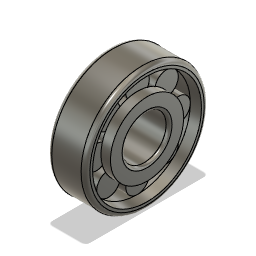
Bearing_GOST_8328-75_12000 (Autodesk Fusion 360 design; units mm, degrees)
Autodesk Fusion 360 part; units mm, degrees
sketch "Sketch1" plane through (0, 0, 0) normal (0, 0, 1) x (1, 0, 0)
  line L0 (-41.4222, 0) -> (41.4222, 0)
  line L1 (-6.5, 7.5) -> (6.5, 7.5)
  line L2 (6.5, 7.5) -> (6.5, 12.4792)
  line L3 (6.5, 12.4792) -> (3.25, 12.4792)
  line L4 (3.25, 12.4792) -> (3.25, 10)
  line L5 (3.25, 10) -> (-3.25, 10)
  line L6 (-3.25, 10) -> (-3.25, 12.4792)
  line L7 (-3.25, 12.4792) -> (-6.5, 12.4792)
  line L8 (-6.5, 12.4792) -> (-6.5, 7.5)
  line L9 (-6.5, 16.5) -> (-6.5, 21)
  line L10 (-6.5, 21) -> (6.5, 21)
  line L11 (6.5, 21) -> (6.5, 18.5731)
  line L12 (6.5, 18.5731) -> (3.25, 18)
  line L13 (3.25, 18) -> (-3.25, 18)
  line L14 (-3.25, 18) -> (-3.25, 16.5)
  line L15 (-3.25, 16.5) -> (-6.5, 16.5)
  line L16 (-3.25, 16.5) -> (-3.25, 12.4792)
  line L17 (3.25, 18) -> (3.25, 12.4792)
  line L18 (0, 18) -> (0, 10) construction
  line L19 (-3.25, 14) -> (3.25, 14)
  point P0 (0, 7.5)
  point P1 (0, 14)
  dimension "d1" = 15
  dimension "d2" = 13
  dimension "d3" = 10
  dimension "d4" = 42
  dimension "d5" = 3.25
  dimension "d6" = 24.9585
  dimension "d7" = 20
  dimension "d8" = 33
  dimension "d9" = 36
  constraint horizontal L0
  constraint midpoint L0 origin
  constraint horizontal L1
  constraint perpendicular L1 L2
  constraint perpendicular L2 L3
  constraint perpendicular L3 L4
  constraint perpendicular L4 L5
  constraint perpendicular L3 L6
  constraint perpendicular L6 L7
  constraint perpendicular L1 L8
  constraint equal L3 L7
  constraint equal L4 L6
  constraint midpoint L1 P0
  constraint vertical origin P0
  constraint vertical L9
  constraint perpendicular L9 L10
  constraint perpendicular L10 L11
  constraint perpendicular L11 L13
  constraint perpendicular L13 L14
  constraint perpendicular L9 L15
  constraint vertical L2.end L11.end
  constraint vertical L7.end L9.start
  constraint vertical L6.end L14.end
  constraint vertical L3.end L12.end
  constraint midpoint L13 L18.start
  constraint perpendicular L13 L18
  constraint midpoint L18 P1
  constraint coincident L5 L18.end
  constraint coincident L16 L19.start
  constraint coincident L17 L19.end
  constraint perpendicular L17 L19
  constraint coincident P1 L19
  measures "d2" distance of L2 L8
  measures "d3" angle of L12 L13
  measures "d5" distance of L2.end L3.end
revolve "Revolve1" add sketch "Sketch1" angle 360 about axis through (-41.4222, 0, 0) along (1, 0, 0) contours L1 L2 L3 L4 L5 L6 L7 L8 | L9 L10 L11 L12 L13 L14 L15 makes body 1 at (-2.1667, 20.8956, -2.0909) makes body 2 at (-2.1667, 7.4627, -0.7468)
revolve "Revolve2" add sketch "Sketch1" angle 360 about axis through (-3.25, 14, 0) along (1, 0, 0) separate body contours L13 L14 L16 L17 L19 makes body 3
pattern_circular "C-Pattern1" count 8 over 360 about axis through (-41.4222, 0, 0) along (1, 0, 0) of bodies 3 makes body 4 at (1.0833, 12.9955, 12.4322) makes body 5 at (1.0833, 0.3983, 17.9801) makes body 6 at (1.0833, -12.4322, 12.9955) makes body 7 at (1.0833, -17.9801, 0.3983) makes body 8 at (1.0833, -12.8654, -12.5834) makes body 9 at (1.0833, -0.3983, -17.9801) makes body 10 at (1.0833, 12.4322, -12.9955)
fillet "Fillet1" radius 1 2 edges at (6.5, -2.7121, 6.9925) (-6.5, -2.7121, 6.9925) on bodies 2
fillet "Fillet2" radius 1.5 2 edges at (6.5, -7.5939, 19.5789) (-6.5, -7.5939, 19.5789) on bodies 1
equation "d5 = ( 13 * 0.25 ) * 1 mm"
